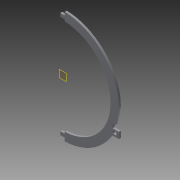
# Autodesk Inventor part: MiddleHoop
Saved by Autodesk Inventor 2013 (Build 170138000, 138)
## iProperties
Created: 2013-01-18
Part Number: MiddleHoop
Material: Generic
Document SubType Name: Modeling
Designer: motoennies
Density: 1 g/cm^3
Author: motoennies
Autodesk Inventor part; units mm, degrees
ref_plane "YZ Plane" through (0, 0, 0) normal (1, 0, 0) x (0, 1, 0)
ref_plane "XZ Plane" through (0, 0, 0) normal (0, 1, 0) x (-1, 0, 0)
ref_plane "XY Plane" through (0, 0, 0) normal (0, 0, 1) x (1, 0, 0)
sketch "Sketch1" plane through (0, 0, 0) normal (0, 0, 1) x (1, 0, 0)
  arc A0 (0, -146.05) -> (0, 146.05) centre (0, 0) ccw
  line L0 (0, 0) -> (0, 226.0912) construction
  line L1 (0, 226.0912) -> (0, -237.3269) construction
  line L2 (6.35, 145.9119) -> (6.35, 171.3324)
  line L3 (6.35, -145.9119) -> (6.35, -171.3324)
  line L4 (0, 146.05) -> (0, 151.13)
  line L5 (0, 151.13) -> (6.35, 151.13)
  line L6 (6.35, 151.13) -> (-7.62, 151.13)
  line L7 (-7.62, 151.13) -> (-7.62, 161.29)
  line L8 (-7.62, 161.29) -> (6.35, 161.29)
  line L9 (0, -146.05) -> (0, -151.13)
  line L10 (0, -151.13) -> (6.35, -151.13)
  line L11 (6.35, -151.13) -> (-7.62, -151.13)
  line L12 (-7.62, -151.13) -> (-7.62, -161.29)
  line L13 (-7.62, -161.29) -> (6.35, -161.29)
  line L14 (171.45, 0) -> (171.45, -82.55)
  line L15 (171.45, -82.55) -> (150.2684, -82.55)
  arc A1 (0, -171.45) -> (150.2684, -82.55) centre (0, 0) ccw
  arc A2 (171.45, 0) -> (0, 171.45) centre (0, 0) ccw
  dimension "d20" = 292.1
  dimension "d21" = 6.35
  dimension "d22" = 6.35
  dimension "d23" = 5.08
  dimension "d24" = 13.97
  dimension "d25" = 10.16
  dimension "d26" = 5.08
  dimension "d27" = 13.97
  dimension "d28" = 10.16
  dimension "d29" = 82.55
  dimension "d45" = 171.45
  dimension "d46" = 171.45
  constraints: 32 end point, 11 point on line, 10 point on circle, 8 perpendicular, 3 centre point, 3 collinear, 3 vertical, 1 coincident, 1 parallel, 1 tangent
  measures "d20" diameter of A0
  measures "d21" distance between parallel lines of L0 L2
  measures "d22" distance between parallel lines of L1 L3
  measures "d23" distance of L4.start L4.end
  measures "d24" distance of L5.end L6.end
  measures "d25" distance of L6.end L7.end
  measures "d26" distance of L9.start L9.end
  measures "d27" distance of L10.end L11.end
  measures "d28" distance of L11.end L12.end
  measures "d29" distance of L14.start L14.end
  measures "d45" radius of A1
  measures "d46" radius of A2
ref_plane "Work Plane1" through (0, 0, 6.35) normal (0, 0, 1) x (1, 0, 0)
sketch "Sketch2" plane through (0, 0, 6.35) normal (0, 0, 1) x (1, 0, 0)
  line L0 (171.45, -82.55) -> (171.45, 0) projected
  line L1 (171.45, -82.55) -> (171.45, -77.0382) construction
  line L2 (171.45, -77.0382) -> (163.83, -77.0382) construction
  line L3 (163.83, -77.0382) -> (153.67, -77.0382)
  line L4 (153.67, -77.0382) -> (153.67, -67.5132)
  line L5 (153.67, -67.5132) -> (163.83, -67.5132)
  line L6 (163.83, -67.5132) -> (163.83, -77.0382)
  line L7 (171.45, 0) -> (171.45, -63.5) construction
  line L8 (171.45, -63.5) -> (152.4, -63.5)
  line L9 (152.4, -63.5) -> (152.4, -50.8)
  line L10 (152.4, -50.8) -> (160.5643, -50.8)
  arc A0 (171.45, 0) -> (6.35, 171.3324) centre (0, 0) ccw projected
  line L11 (160.5643, -50.8) -> (171.45, 0)
  line L12 (171.45, 0) -> (171.45, -63.5)
  point P0 (171.45, -44.45)
  dimension "d32" = 5.5118
  dimension "d33" = 7.62
  dimension "d34" = 10.16
  dimension "d35" = 9.525
  dimension "d38" = 63.5
  dimension "d39" = 19.05
  dimension "d40" = 12.7
  dimension "d44" = 102.095
  constraints: 24 end point, 5 perpendicular, 3 point on line, 2 collinear, 2 parallel, 1 point on circle, 1 tangent
  measures "d32" distance of L0.start L1.end
  measures "d33" distance of L1.end L2.end
  measures "d34" distance of L2.end L3.end
  measures "d35" distance of L3.end L4.end
  measures "d38" distance of L0.end L7.end
  measures "d39" distance of L7.end L8.end
  measures "d40" distance of L8.end L9.end
  measures "d44" angle of L11 L10
extrude "Extrusion5" add sketch "Sketch1" along normal blind 6.35 contours A0 L2 A2 L14 L15 A1 L3 | L10 L3 L13 L12 L11 | L5 L6 L7 L8 L2
extrude "Extrusion6" cut sketch "Sketch2" against normal blind 6.35
body "Solid2"
